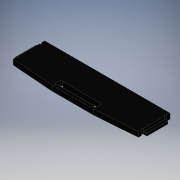
# Autodesk Inventor part: コックピット_サブフレーム_1_6
Saved by Autodesk Inventor 2018 (Build 220112000, 112)
## iProperties
Created: 2016-05-09
Part Number: コックピット_サブフレーム_1_6
Material: アセタール樹脂、黒
Document SubType Name: Modeling
Designer: hiroaki
Density: 1.425 g/cm^3
Appearance: 滑らか - 黒
Mass: 13.4294 g
Surface Area: 78.6855 cm^2
Volume: 9.42414 cm^3
Author: hiroaki
Autodesk Inventor part; units mm, degrees
ref_plane "YZ Plane" through (0, 0, 0) normal (1, 0, 0) x (0, 1, 0)
ref_plane "XZ Plane" through (0, 0, 0) normal (0, 1, 0) x (-1, 0, 0)
ref_plane "XY Plane" through (0, 0, 0) normal (0, 0, 1) x (1, 0, 0)
sketch "スケッチ1" plane through (0, 0, 0) normal (0, 0, 1) x (1, 0, 0)
  line L0 (-59.5, -15) -> (59.5, -15) construction
  line L1 (59.5, -15) -> (59.5, 15) construction
  line L2 (59.5, 15) -> (-59.5, 15) construction
  line L3 (-59.5, 15) -> (-59.5, -15) construction
  line L4 (-59.5, -15) -> (59.5, 15) construction
  line L5 (59.5, -15) -> (-59.5, 15) construction
  line L6 (-59.5, 12.1) -> (-59.5, 15)
  line L7 (-59.5, 15) -> (59.5, 15)
  line L8 (59.5, 15) -> (59.5, 12.1)
  line L9 (-59.5, -12.1) -> (-59.5, -15)
  line L10 (59.5, -15) -> (59.5, -12.1)
  line L11 (-59.5, 10) -> (-62.5, 10)
  line L12 (-62.5, 10) -> (-62.5, -10)
  line L13 (-62.5, -10) -> (-59.5, -10)
  arc A0 (-59.5, 10) -> (-59.5, 12.1) centre (-59.5, 11.05) ccw
  line L14 (0, 0) -> (0, 15) construction
  line L15 (0, 0) -> (-59.5, 0) construction
  arc A1 (-59.5, -12.1) -> (-59.5, -10) centre (-59.5, -11.05) ccw
  line L16 (59.5, 10) -> (62.5, 10)
  line L17 (62.5, 10) -> (62.5, -10)
  line L18 (62.5, -10) -> (59.5, -10)
  arc A2 (59.5, 12.1) -> (59.5, 10) centre (59.5, 11.05) ccw
  arc A3 (59.5, -10) -> (59.5, -12.1) centre (59.5, -11.05) ccw
  line L19 (-59.5, -15) -> (-19.5, -18)
  line L20 (-19.5, -18) -> (19.5, -18)
  line L21 (19.5, -18) -> (59.5, -15)
  line L22 (-19.5, -10) -> (19.5, -10) construction
  line L23 (19.5, -10) -> (19.5, -15) construction
  line L24 (19.5, -15) -> (-19.5, -15) construction
  line L25 (-19.5, -15) -> (-19.5, -10) construction
  line L26 (19.55, -9.95) -> (-19.55, -9.95)
  line L27 (-19.55, -9.95) -> (-19.55, -15.05)
  line L28 (-19.55, -15.05) -> (19.55, -15.05)
  line L29 (19.55, -15.05) -> (19.55, -9.95)
  circle A4 centre (-18.5, -9.95) radius 1.05
  circle A5 centre (-18.5, -15.05) radius 1.05
  circle A6 centre (18.5, -9.95) radius 1.05
  circle A7 centre (18.5, -15.05) radius 1.05
  dimension "d9" = 2.1
  dimension "d0" = 119
  dimension "d1" = 30
  dimension "d2" = 1.05
  dimension "d3" = 20
  dimension "d4" = 3
  dimension "d5" = 5
  dimension "d6" = 0.05
  dimension "d7" = 39
  dimension "d8" = 3
  constraints: 60 end point, 9 perpendicular, 8 point on circle, 6 collinear, 6 parallel, 6 vertical alignment, 5 horizontal, 4 centre point, 4 horizontal alignment, 4 midpoint, 4 point on line, 4 tangent, 3 equal radius, 2 symmetric about line, 2 vertical, 15 other
  measures "d0" distance of L1.end L2.end
  measures "d1" distance of L0.end L1.end
  measures "d2" radius of A0
  measures "d3" distance of L11.end L12.end
  measures "d4" distance between parallel lines of L3 L12
  measures "d5" distance of L24.end L22.start
  measures "d6" distance between parallel lines of L26 L22
  measures "d7" distance of L22.start L22.end
  measures "d8" distance between parallel lines of L20 L0
extrude "押し出し1" add sketch "スケッチ1" along normal blind 5
sketch "スケッチ2" plane through (0, 0, 5) normal (0, 0, 1) x (1, 0, 0)
  line L0 (59.5, 12.1) -> (59.5, 15) projected
  line L1 (-59.5, 15) -> (-59.5, 12.1) projected
  line L2 (65.6261, 13.972) -> (59.5, 13.972)
  line L3 (59.5, 13.972) -> (59.5, -16.1)
  line L4 (59.5, -16.1) -> (65.6261, -16.1)
  line L5 (65.6261, -16.1) -> (65.6261, 13.972)
  line L6 (-65.8886, -16.1) -> (-59.5, -16.1)
  line L7 (-59.5, -16.1) -> (-59.5, 18.3327)
  line L8 (-59.5, 18.3327) -> (-65.8886, 18.3327)
  line L9 (-65.8886, 18.3327) -> (-65.8886, -16.1)
  point P0 (0, 0)
  constraints: 16 end point, 4 parallel, 2 collinear, 2 horizontal, 2 perpendicular, 1 point on line
extrude "押し出し2" cut sketch "スケッチ2" against normal blind 2.5
